Steckerhalter Anhnger Norbert (Autodesk Fusion 360 design; units mm, degrees)
Autodesk Fusion 360 part; units mm, degrees
sketch "Sketch1" plane through (0, 0, 0) normal (0, 1, 0) x (1, 0, 0)
  line L0 (0, 0) -> (100, 0)
  line L1 (100, 0) -> (100, -100)
  line L2 (100, -100) -> (0, -100)
  line L3 (0, -100) -> (0, 0)
  dimension "d1" = 100
  dimension "d2" = 100
  constraint horizontal L0
  constraint vertical L1
  constraint horizontal L2
  constraint vertical L3
  constraint coincident L0.start L3.end
  measures "d1" distance of L0.start L0.end
  measures "d2" distance of L0.start L2.end
sketch "Sketch2" plane through (0, 0, 0) normal (0, 1, 0) x (1, 0, 0)
  circle A0 centre (19, -57) radius 22.5
  circle A1 centre (5.9292, -79.3772) radius 5
  circle A2 centre (45.3, -57.3) radius 5
  circle A3 centre (6.4, -34.3) radius 5
  circle A4 centre (45.3, -57.3) radius 1.5
  circle A5 centre (5.9292, -79.3772) radius 1.5
  circle A6 centre (6.4, -34.3) radius 1.5
  line L0 (6.4, -34.3) -> (45.3, -57.3)
  line L1 (45.3, -57.3) -> (50.0703, -49.232)
  line L2 (50.0703, -49.232) -> (11.1703, -26.232)
  line L3 (11.1703, -26.232) -> (6.4, -34.3)
  line L4 (34.4579, -50.8895) -> (17.2421, -40.7105)
  line L5 (17.2421, -40.7105) -> (22.0124, -32.6424)
  line L6 (22.0124, -32.6424) -> (39.2282, -42.8215)
  line L7 (39.2282, -42.8215) -> (34.4579, -50.8895)
  point P0 (45.3, -57.3)
  point P1 (30.6203, -37.732)
  dimension "d3" = 45
  dimension "d4" = 10
  dimension "d5" = 10
  dimension "d6" = 10
  dimension "d7" = 3
  dimension "d8" = 3
  dimension "d9" = 3
  dimension "d17" = 20
  constraint coincident P0 A2.centre
  constraint coincident A1.centre A5.centre
  constraint coincident A3.centre A6.centre
  constraint perpendicular L0 L1
  constraint parallel L0 L2
  constraint parallel L1 L3
  constraint tangent A0 L2
  constraint perpendicular L4 L5
  constraint parallel L4 L6
  constraint parallel L5 L7
  constraint coincident L0 L4.end
  constraint parallel L0 L4
  constraint midpoint L2 P1
  constraint midpoint L6 P1
  measures "d3" diameter of A0
  measures "d4" diameter of A1
  measures "d5" diameter of A2
  measures "d6" diameter of A3
  measures "d7" diameter of A4
  measures "d8" diameter of A5
  measures "d9" diameter of A6
  measures "d17" distance of L5.end L6.end
extrude "Extrude1" add sketch "Sketch2" along normal blind 5 contours A0 A2 L0 | A0 A2 A4 L0 L1 | A0 A2 L0 | A0 A2 A4 L0 L1 | A0 A1 A2 A3 L0 L4 | A0 A2 L0 L7 | A0 A1 | A0 A1 | A0 L0 L4 L5 L7 | A0 A3 L0 L5 | A0 A3 A6 L0 L3 | A0 A3 L0 | A0 A3 L0 | A0 A3 A6 L0 L3
fillet "Fillet1" radius 11 6 edges at (41.3322, 2.5, 54.2575) (11.1298, 2.5, 35.9213) (41.2639, 2.5, 60.2512) (10.7114, 2.5, 77.9177) (4.8513, 2.5, 74.4947) (5.2742, 2.5, 39.1716)
extrude "Extrude2" add sketch "Sketch2" along normal blind 5 contours A0 A2 L1 L2 L7 | A0 L2 L6 L7 | A0 L2 L5 L6 | A0 A3 L2 L3 L5
extrude "Extrude3" add sketch "Sketch2" along normal blind 20 contours A0 L0 L4 L5 L7 | A0 L2 L6 L7 | A0 L2 L5 L6
sketch "Sketch4" plane through (-8.5988, 0, 14.5433) normal (0.508953, 0, -0.860794) x (0, 1, 0)
  line L0 (5, 55.5616) -> (5, 68.157)
  line L1 (5, 68.157) -> (0, 68.157)
  line L2 (0, 68.157) -> (0, 22.9662)
  line L3 (0, 22.9662) -> (5, 22.9662)
  line L4 (5, 22.9662) -> (5, 35.5616)
  line L5 (5, 35.5616) -> (20, 35.5616)
  line L6 (20, 35.5616) -> (20, 55.5616)
  line L7 (20, 55.5616) -> (5, 55.5616)
  circle A0 centre (12, 45.5616) radius 2.5
  line L8 (20, 45.5616) -> (-11, 45.5616)
  point P0 (20, 45.5616)
  point P1 (-8.5888, 45.5616)
  dimension "d20" = 5
  dimension "d21" = 8
  constraint midpoint L6 P0
  constraint coincident P0 L8.start
  constraint perpendicular L6 L8
  constraint coincident A0.centre L8
  measures "d20" diameter of A0
  measures "d21" distance of L6 A0.centre
extrude "Extrude4" cut sketch "Sketch4" against normal blind 16 contours A0 L8 | A0 L8
fillet "Fillet2" radius 18 2 edges at (50.0703, 2.5, 49.232) (11.1703, 2.5, 26.232)
fillet "Fillet3" radius 39.5 2 edges at (8.9448, 2.5, 29.996) (47.8448, 2.5, 52.996)
fillet "Fillet4" radius 8.5 2 edges at (36.8431, 5, 46.8555) (19.6272, 5, 36.6765)
fillet "Fillet5" radius 5.5 1 edges at (25.85, 5, 45.8)
